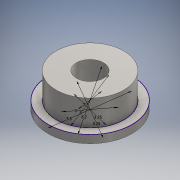
# Autodesk Inventor part: ベアリング
Saved by Autodesk Inventor 2016 (Build 200138000, 138)
## iProperties
Created: 2016-12-02
Part Number: ベアリング
Material: 一般
Document SubType Name: Modeling
Designer: KOTA-NPC2
Density: 1 g/cm^3
Appearance: ステンレス - ブラシ仕上げ
Author: KOTA-NPC2
Autodesk Inventor part; units mm, degrees
ref_plane "YZ Plane" through (0, 0, 0) normal (1, 0, 0) x (0, 1, 0)
ref_plane "XZ Plane" through (0, 0, 0) normal (0, 1, 0) x (-1, 0, 0)
ref_plane "XY Plane" through (0, 0, 0) normal (0, 0, 1) x (1, 0, 0)
sketch "スケッチ1" plane through (0, 0, 0) normal (0, 0, 1) x (1, 0, 0)
  circle A0 centre (0, 0) radius 3.1
  circle A1 centre (0, 0) radius 2.5
  circle A2 centre (0, 0) radius 1
  dimension "d0" = 6.2
  dimension "d1" = 5
  dimension "d2" = 2
  constraints: 3 centre point, 3 coincident
  measures "d0" diameter of A0
  measures "d1" diameter of A1
  measures "d2" diameter of A2
extrude "押し出し1" add sketch "スケッチ1" against normal blind 0.6 contours A0 | A1
extrude "押し出し2" add sketch "スケッチ1" along normal blind 1.9 contours A1
sketch "スケッチ2" plane through (0, 0, -0.6) normal (0, 0, -1) x (-1, 0, 0)
  circle A0 centre (0, 0) radius 2.75
  circle A1 centre (0, 0) radius 1.5
  circle A2 centre (0, 0) radius 2.625
  circle A3 centre (0, 0) radius 1.625
  dimension "d7" = 5.5
  dimension "d8" = 3
  dimension "d11" = 5.25
  dimension "d12" = 3.25
  constraints: 4 centre point, 4 coincident
  measures "d7" diameter of A0
  measures "d8" diameter of A1
  measures "d11" diameter of A2
  measures "d12" diameter of A3
extrude "押し出し4" cut sketch "スケッチ2" against normal blind 0.5 contours A3
extrude "押し出し5" cut sketch "スケッチ2" against normal blind 0.5 contours A0
